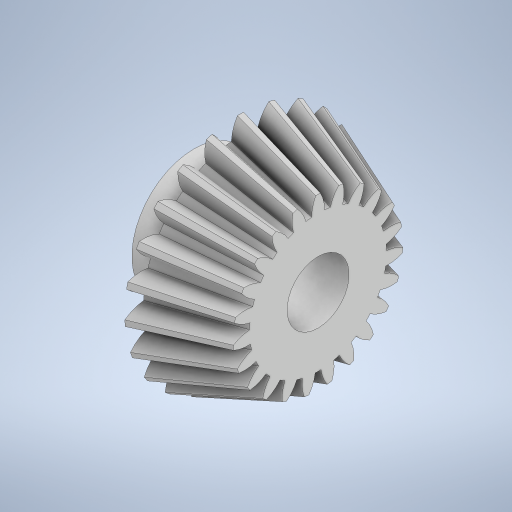
# Autodesk Inventor part: bevel
Saved by Autodesk Inventor 2024 (Build 280153000, 153)
## iProperties
Created: 2023-05-14
Part Number: bevel
Material: Generic
Document SubType Name: Modeling
Designer: shraa
Density: 1 g/cm^3
Appearance: Default
Author: shraa
Autodesk Inventor part; units mm, degrees
ref_plane "YZ Plane" through (0, 0, 0) normal (1, 0, 0) x (0, 1, 0)
ref_plane "XZ Plane" through (0, 0, 0) normal (0, 1, 0) x (-1, 0, 0)
ref_plane "XY Plane" through (0, 0, 0) normal (0, 0, 1) x (1, 0, 0)
sketch "Sketch1" plane through (0, 0, 0) normal (0, 0, 1) x (1, 0, 0)
  line L0 (0, 0) -> (0, 20)
  line L1 (0, 20) -> (10, 20)
  line L2 (15, 25) -> (15, 31.16)
  line L3 (15, 31.16) -> (100.6114, 0)
  line L4 (100.6114, 0) -> (0, 0)
  arc A0 (10, 20) -> (15, 25) centre (10, 25) ccw
  line L5 (40, 22.0607) -> (40, 0)
  line L6 (0, 10) -> (40, 10)
  point P0 (15, 20)
  point P1 (15, 28.08)
  dimension "d0" = 15
  dimension "d1" = 40
  dimension "d2" = 62.32
  dimension "d3" = 20
  dimension "d4" = 5
  dimension "d5" = 25
  dimension "d6" = 20
  constraints: 14 end point, 5 point on line, 4 perpendicular, 2 midpoint, 2 point on circle, 2 tangent, 2 vertical, 1 centre point
  measures "d0" distance of L0.end point (15, 20)
  measures "d1" diameter of L1 L4
  measures "d2" diameter of L2.end L4
  measures "d3" angle of L3 L4
  measures "d4" radius of A0
  measures "d5" distance from line of point (15, 28.08) L5
  measures "d6" diameter of L6 L4
revolve "Revolution1" add sketch "Sketch1" angle 360 about axis through (100.6114, 0, 0) along (-1, 0, 0) contours L0 L1 A0 L2 L3 L5 L6
sketch "Sketch2" plane through (40, 0, 0) normal (1, 0, 0) x (0, 0, -1)
  circle A0 centre (0, 0) radius 22.0607 construction
  arc A1 (2.08, 21.9625) -> (-2.08, 21.9625) centre (0, 0) ccw
  arc A2 (0.745, 27.3148) -> (-0.745, 27.3148) centre (0, 0) ccw
  arc A3 (-0.745, 27.3148) -> (-2.08, 21.9625) centre (9.1599, 22.0017) ccw
  arc A4 (2.08, 21.9625) -> (0.745, 27.3148) centre (-9.1599, 22.0017) ccw
  dimension "d8" = 4.16
  dimension "d9" = 2.08
  dimension "d10" = 27.325
  dimension "d11" = 0.745
  dimension "d12" = 1.49
  dimension "d13" = 11.24
  dimension "d14" = 11.24
  constraints: 10 point on circle, 4 centre point, 2 coincident
  measures "d8" distance of A0.start A0.end
  measures "d9" horizontal distance of point (0, 0) A0.end
  measures "d10" radius of A2
  measures "d11" horizontal distance of A2.end point (0, 0)
  measures "d12" distance of A2.end A2.start
  measures "d13" radius of A3
  measures "d14" radius of A4
sketch "Sketch3" plane through (15, 0, 0) normal (-1, 0, 0) x (0, 0, 1)
  circle A0 centre (0, 0) radius 31.16 projected
  arc A1 (2.915, 31.0234) -> (-2.915, 31.0234) centre (0, 0) ccw construction
  circle A2 centre (0, 0) radius 20 projected
  arc A3 (0.975, 37.2672) -> (-0.975, 37.2672) centre (0, 0) ccw
  arc A4 (-0.975, 37.2672) -> (-2.915, 31.0234) centre (9.2101, 30.6794) ccw
  arc A5 (2.915, 31.0234) -> (0.975, 37.2672) centre (-9.2101, 30.6794) ccw
  dimension "d15" = 2.915
  dimension "d16" = 5.83
  dimension "d18" = 37.28
  dimension "d19" = 0.975
  dimension "d20" = 1.95
  dimension "d21" = 12.13
  dimension "d22" = 12.13
  constraints: 10 point on circle, 4 centre point, 2 coincident, 1 concentric
  measures "d15" horizontal distance of point (0, 0) A0.end
  measures "d16" distance of A0.end A0.start
  measures "d18" radius of A3
  measures "d19" horizontal distance of point (0, 0) A3.end
  measures "d20" distance of A3.end A3.start
  measures "d21" radius of A4
  measures "d22" radius of A5
loft "Loft1" add profiles "Sketch2", "Sketch3" contours all / A0 A4 A3 A5
pattern_circular "Circular Pattern1" count 23 over 360 about axis through (20, 0, 0) along (-1, 0, 0) of "Loft1"
sketch "Sketch4" plane through (0, 0, 0) normal (-1, 0, 0) x (0, 0, 1)
  point P0 (0, 0)
body "Solid1"
